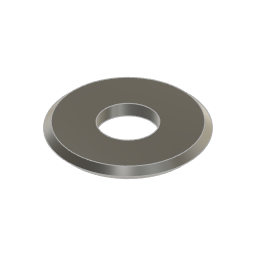
Washer (Autodesk Fusion 360 design; units mm, degrees)
Autodesk Fusion 360 part; units mm, degrees
sketch "Sketch1" plane through (0, 0, 0) normal (0, 0, 1) x (1, 0, 0)
  circle A0 centre (0, 0) radius 26.1874
  circle A1 centre (0, 0) radius 9.906
  dimension "d1" = 52.3748
  dimension "d2" = 19.812
  constraint coincident A0.centre A1.centre
  constraint concentric A0 A1
  measures "d1" diameter of A0
  measures "d2" diameter of A1
extrude "Extrude1" add sketch "Sketch1" along normal blind 4.7498
chamfer "Chamfer1" distance 2.3622 angle 45 2 edges at (-24.4152, -9.4698, 4.7498) (-24.4152, -9.4698, 0)
